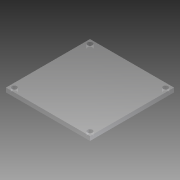
# Autodesk Inventor part: 13_0204_004-1
Saved by Autodesk Inventor 2012 SP1 (Build 160190100, 190)
## iProperties
Created: 2013-03-21
Part Number: 13_0204_004-1
Material: Default
Document SubType Name: Modeling
Designer: vogel
Density: 1 g/cm^3
Author: vogel
Autodesk Inventor part; units mm, degrees
ref_plane "YZ Plane" through (0, 0, 0) normal (1, 0, 0) x (0, 1, 0)
ref_plane "XZ Plane" through (0, 0, 0) normal (0, 1, 0) x (-1, 0, 0)
ref_plane "XY Plane" through (0, 0, 0) normal (0, 0, 1) x (1, 0, 0)
sketch "Skizze1" plane through (0, 0, 0) normal (0, 0, 1) x (1, 0, 0)
  line L0 (0, 0) -> (40, 0)
  line L1 (40, 0) -> (40, 40)
  line L2 (40, 40) -> (0, 40)
  line L3 (0, 40) -> (0, 0)
  dimension "d0" = 40
  dimension "d1" = 40
  constraints: 8 end point, 2 parallel, 1 horizontal, 1 perpendicular
  measures "d0" distance of L2.end L0.start
  measures "d1" distance of L0.start L0.end
extrude "Extrusion1" add sketch "Skizze1" along normal blind 2
sketch "Skizze3" plane through (0, 0, 2) normal (0, 0, 1) x (1, 0, 0)
  line L0 (0, 0) -> (0, 40) projected
  line L1 (40, 0) -> (0, 0) projected
  line L2 (40, 40) -> (40, 0) projected
  line L3 (0, 40) -> (40, 40) projected
  line L4 (36, 36) -> (36, 4)
  line L5 (36, 4) -> (4, 4)
  line L6 (4, 4) -> (4, 36)
  line L7 (4, 36) -> (36, 36)
  line L8 (38, 38) -> (38, 2)
  line L9 (38, 2) -> (2, 2)
  line L10 (2, 2) -> (2, 38)
  line L11 (2, 38) -> (38, 38)
  dimension "d14" = 4
  dimension "d15" = 2
  constraints: 16 end point, 4 coincident, 6 other
  measures "d14" distance between parallel lines of L3 L7
  measures "d15" distance between parallel lines of L3 L11
hole "Bohrung2" at (38, 38, 2) at (2, 38, 2) at (2, 2, 2) at (38, 2, 2) direction (0, 0, -1) diameter 2.4 end through all
